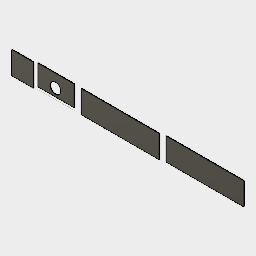
Auto Teile Wand (Autodesk Fusion 360 design; units mm, degrees)
Autodesk Fusion 360 part; units mm, degrees
sketch "Skizze2" plane through (0, 0, 0) normal (0, 1, 0) x (1, 0, 0)
box "Grundkörper Quader5" add length 70 width 40 height 1 placed x (0, 1, 0) y (-1, 0, 0) z (0, 0, 1) at (9840, -1100, 0) makes body 1
hole "Bohrung2" at (9814.7296, -1063.7243, 0) direction (0, 0, 1) diameter 20 depth 30 tip angle 118 bodies 1
move_body "Verschieben4" bodies 1 to x (0, 1, 0) y (-1, 0, 0) z (0, 0, 1) at (8795, -10855, 0)
box "Grundkörper Quader6" add length 42 width 44 height 1 placed x (0, 1, 0) y (-1, 0, 0) z (0, 0, 1) at (9815, -1050, 0) separate body makes body 2
move_body "Verschieben5" bodies 2 to x (0, 1, 0) y (-1, 0, 0) z (0, 0, 1) at (8745, -10845, 0)
move_body "Verschieben6" bodies 2 to x (1, 0, 0) y (0, 1, 0) z (0, 0, 1) at (23.8524, 14.6956, 2.3493)
box "Grundkörper Quader7" add length 44 width 150 height 1 placed x (0, -1, 0) y (1, 0, 0) z (0, 0, 1) at (9908.5893, -1015.7698, 0) separate body makes body 3
copy_body "Körper kopieren/einfügen1" bodies 3 makes body 4
move_body "Verschieben7" bodies 4 to x (1, 0, 0) y (0, 1, 0) z (0, 0, 1) at (79.9205, 0, -172.6733)
move_body "Verschieben8" bodies 4 to x (1, 0, 0) y (0, 1, 0) z (0, 0, 1) at (80, 0, 170)
